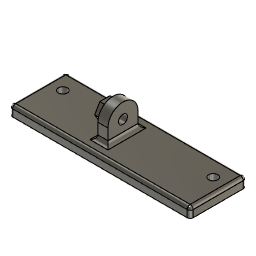
Camera Stand Part 1 (Autodesk Fusion 360 design; units mm, degrees)
Autodesk Fusion 360 part; units mm, degrees
note: some values were not read from the file. Set by a fixed rule: the direction of a hole.
sketch "Sketch1" plane through (0, 0, 0) normal (0, 0, 1) x (1, 0, 0)
  line L0 (-45, 14) -> (45, 14)
  line L1 (45, 14) -> (45, -14)
  line L2 (45, -14) -> (-45, -14)
  line L3 (-45, -14) -> (-45, 14)
  line L4 (-45, 14) -> (45, -14) construction
  line L5 (45, 14) -> (-45, -14) construction
  dimension "d1" = 90
  dimension "d2" = 28
  constraint horizontal L0
  constraint perpendicular L0 L1
  constraint parallel L0 L2
  constraint parallel L1 L3
  constraint coincident L4 origin
  constraint coincident L5 origin
  measures "d1" distance of L1.end L2.end
  measures "d2" distance of L0.end L1.end
extrude "Extrude1" add sketch "Sketch1" along normal blind 5
sketch "Sketch2" plane through (0, 0, 0) normal (0, 0, 1) x (1, 0, 0)
  line L0 (0, 0) -> (37.5, 0)
  line L1 (0, 0) -> (-37.5, 0)
  circle A0 centre (37.5, 0) radius 2
  circle A1 centre (-37.5, 0) radius 2
  dimension "d5" = 37.5
  dimension "d6" = 37.5
  dimension "d7" = 4
  dimension "d8" = 4
  constraint coincident L0.start L1.start
  constraint horizontal L0
  constraint parallel L0 L1
  constraint coincident L0.end A0.centre
  constraint coincident L1.end A1.centre
  measures "d5" distance of L0.start L0.end
  measures "d6" distance of L0.start L1.end
  measures "d7" diameter of A0
  measures "d8" diameter of A1
sketch "Sketch3" plane through (0, 0, 0) normal (0, 0, 1) x (1, 0, 0)
  line L0 (0, 0) -> (-37.5, 0)
  circle A0 centre (-37.5, 0) radius 2
  dimension "d11" = 37.5
  dimension "d12" = 4
  constraint coincident L0.start origin
  constraint horizontal L0
  constraint coincident L0.end A0.centre
  measures "d11" distance of L0.start L0.end
  measures "d12" diameter of A0
ref_plane "WorkPlane1" through (0, 0, 5) normal (0, 0, 1) x (1, 0, 0)
sketch "Sketch4" plane through (0, 0, 5) normal (0, 0, 1) x (1, 0, 0)
  line L0 (0, 0) -> (-5, 0)
  line L1 (-2.5, 7.5) -> (-7.5, 7.5)
  line L2 (-7.5, 7.5) -> (-7.5, -7.5)
  line L3 (-7.5, -7.5) -> (-2.5, -7.5)
  line L4 (-2.5, -7.5) -> (-2.5, 7.5)
  line L5 (-2.5, 7.5) -> (-7.5, -7.5) construction
  line L6 (-7.5, 7.5) -> (-2.5, -7.5) construction
  point P0 (-5, 0)
  dimension "d16" = 5
  dimension "d17" = 5
  dimension "d18" = 15
  constraint coincident L0.start origin
  constraint horizontal L0
  constraint horizontal L1
  constraint perpendicular L1 L2
  constraint parallel L1 L3
  constraint parallel L2 L4
  constraint coincident L5 P0
  constraint coincident L6 P0
  constraint coincident P0 L0.end
  measures "d16" distance of L0.start P0
  measures "d17" distance of L2.end L3.end
  measures "d18" distance of L1.end L2.end
extrude "Extrude4" add sketch "Sketch4" along normal blind 15
sketch "Sketch5" plane through (0, 0, 5) normal (0, 0, 1) x (-1, 0, 0)
  line L0 (2.5, 7.5) -> (7.5, 7.5)
  line L1 (7.5, 7.5) -> (7.5, -7.5)
  line L2 (7.5, -7.5) -> (2.5, -7.5)
  line L3 (2.5, -7.5) -> (2.5, 7.5)
  line L4 (45, 14) -> (-45, 14)
  line L5 (-45, 14) -> (-45, -14)
  line L6 (-45, -14) -> (45, -14)
  line L7 (45, -14) -> (45, 14)
  line L8 (0, 0) -> (-5, 0)
  line L9 (-7.5, -7.5) -> (-2.5, -7.5)
  line L10 (-2.5, -7.5) -> (-2.5, 7.5)
  line L11 (-2.5, 7.5) -> (-7.5, 7.5)
  line L12 (-7.5, 7.5) -> (-7.5, -7.5)
  line L13 (-7.5, -7.5) -> (-2.5, 7.5) construction
  line L14 (-2.5, -7.5) -> (-7.5, 7.5) construction
  point P0 (-5, 0)
  dimension "d23" = 5
  dimension "d24" = 5
  dimension "d25" = 15
  constraint coincident L8.start origin
  constraint perpendicular L3 L8
  constraint horizontal L9
  constraint perpendicular L9 L10
  constraint parallel L9 L11
  constraint parallel L10 L12
  constraint coincident L13 P0
  constraint coincident L14 P0
  constraint coincident P0 L8.end
  measures "d23" distance of L8.start P0
  measures "d24" distance of L10.end L11.end
  measures "d25" distance of L9.end L10.end
hole "Hole1" at (7.5, 0, 9.3622) direction (-1, 0, 0) diameter 4.5 depth 6 tip angle 118
hole "Hole2" at (-2.5, 0, 12.5) direction (-1, 0, 0) diameter 4.5 depth 6 tip angle 118
fillet "Fillet3" radius 1.5 2 edges at (0, 14, 5) (0, -14, 5)
sketch "Sketch6" plane through (0, 0, 0) normal (0, 0, 1) x (1, 0, 0)
  line L0 (0, 0) -> (37.5, 0)
  line L1 (37.5, 0) -> (37.5, 5)
  line L2 (0, 0) -> (-37.5, 0)
  line L3 (-37.5, 0) -> (-37.5, 5)
  dimension "d38" = 37.5
  dimension "d39" = 5
  dimension "d40" = 37.5
  dimension "d41" = 5
  constraint coincident L0.start L2.start
  constraint horizontal L0
  constraint perpendicular L0 L1
  constraint parallel L0 L2
  constraint perpendicular L2 L3
  measures "d38" distance of L0.start L0.end
  measures "d39" distance of L0.end L1.end
  measures "d40" distance of L0.start L2.end
  measures "d41" distance of L2.end L3.end
hole "Hole3" at (-37.5, 5, 0) direction (0, 0, 1) diameter 4.5 depth 5 tip angle 118
sketch "Sketch7" plane through (0, 0, 0) normal (0, 0, 1) x (1, 0, 0)
  line L0 (0, 0) -> (37.5, 0)
  line L1 (37.5, 0) -> (37.5, 5)
  dimension "d45" = 37.5
  dimension "d46" = 5
  constraint coincident L0.start origin
  constraint horizontal L0
  constraint perpendicular L0 L1
  measures "d45" distance of L0.start L0.end
  measures "d46" distance of L0.end L1.end
hole "Hole4" at (37.5, 5, 0) direction (0, 0, 1) diameter 4.5 depth 5 tip angle 118
fillet "Fillet4" radius 1.5 10 edges at (-45, 14, 1.75) (-45, 13.5607, 4.5607) (-45, 0, 5) (-45, -13.5607, 4.5607) (-45, -14, 1.75) (45, -14, 1.75) (45, -13.5607, 4.5607) (45, 0, 5) (45, 13.5607, 4.5607) (45, 14, 1.75)
fillet "Fillet5" radius 7.5 2 edges at (-5, -7.5, 20) (-5, 7.5, 20)
fillet "Fillet6" radius 2 4 edges at (-5, -7.5, 5) (-2.5, 0, 5) (-5, 7.5, 5) (-7.5, 0, 5)
sketch "Sketch8" plane through (-2.5, 0, 0) normal (1, 0, 0) x (0, 1, 0)
  line L0 (-7.5, 7) -> (7.5, 7)
  line L1 (7.5, 7) -> (7.5, 12.5)
  arc A0 (7.5, 12.5) -> (-7.5, 12.5) centre (0, 12.5) ccw
  line L2 (-7.5, 12.5) -> (-7.5, 7)
  circle A1 centre (0, 12.5) radius 2.25
  line L3 (1.9774, 15.925) -> (-1.9774, 15.925)
  line L4 (-1.9774, 15.925) -> (-3.9548, 12.5)
  line L5 (-3.9548, 12.5) -> (-1.9774, 9.075)
  line L6 (-1.9774, 9.075) -> (1.9774, 9.075)
  line L7 (1.9774, 9.075) -> (3.9548, 12.5)
  line L8 (3.9548, 12.5) -> (1.9774, 15.925)
  line L9 (-5.1095, 12.5) -> (-2.5548, 8.075)
  line L10 (-2.5548, 8.075) -> (2.5548, 8.075)
  line L11 (2.5548, 8.075) -> (5.1095, 12.5)
  line L12 (5.1095, 12.5) -> (2.5548, 16.925)
  line L13 (2.5548, 16.925) -> (-2.5548, 16.925)
  line L14 (-2.5548, 16.925) -> (-5.1095, 12.5)
  point P0 (0, 12.5)
  dimension "d56" = 6.85
  dimension "d57" = 1
  constraint coincident P0 A0.centre
  constraint horizontal L3
  measures "d56" distance of L3 L6
extrude "Extrude6" add sketch "Sketch8" against normal blind 4 from surface at -5 contours L9 L10 L11 L12 L13 L14
